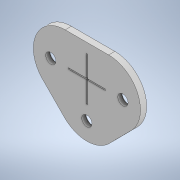
# Autodesk Inventor part: Cover
Saved by Autodesk Inventor 2021 (Build 250183000, 183)
## iProperties
Created: 2021-05-18
Part Number: Cover
Material: Generic
Document SubType Name: Modeling
Designer: Timo
Density: 1 g/cm^3
Appearance: Default
Mass: 1.07498 g
Surface Area: 14.5112 cm^2
Volume: 1.07498 cm^3
Author: Timo
Autodesk Inventor part; units mm, degrees
ref_plane "YZ Plane" through (0, 0, 0) normal (1, 0, 0) x (0, 1, 0)
ref_plane "XZ Plane" through (0, 0, 0) normal (0, 1, 0) x (-1, 0, 0)
ref_plane "XY Plane" through (0, 0, 0) normal (0, 0, 1) x (1, 0, 0)
sketch "Sketch1" plane through (0, 0, 0) normal (0, 0, 1) x (1, 0, 0)
  circle A0 centre (0, 0) radius 6.5 construction
  ellipse E0 centre (0, -17.162) end of major axis (0, -11.841) minor radius 5 construction
  line L0 (0, -44.4052) -> (0, 16.7342) projected
  ellipse E1 centre (0, -19.38) end of major axis (0, -14.059) minor radius 5 construction
  line L1 (0, -17.162) -> (0, -19.38) construction
  line L2 (-6, -17.162) -> (-6, -19.38)
  line L3 (6, -19.38) -> (6, -17.162)
  arc A1 (6, -17.162) -> (-6, -17.162) centre (0, -17.162) ccw
  arc A2 (-6, -19.38) -> (6, -19.38) centre (0, -19.38) ccw
  circle A3 centre (0, 0) radius 8 construction
  circle A4 centre (11.65, -18.271) radius 1.65
  line L4 (11.65, -18.271) -> (6, -18.271) construction
  circle A5 centre (-11.65, -18.271) radius 1.65
  line L5 (7.029, -18.271) -> (-7.029, -18.271) construction
  line L6 (7.029, -28.542) -> (-7.029, -28.542)
  line L7 (-7.029, -8) -> (7.029, -8)
  arc A6 (7.029, -28.542) -> (7.029, -8) centre (7.029, -18.271) ccw
  arc A7 (-7.029, -8) -> (-7.029, -28.542) centre (-7.029, -18.271) ccw
  circle A8 centre (0, -30) radius 1.65
  circle A9 centre (0, -25.4) radius 10.271
  line L8 (-14.3428, -25.4822) -> (-7.3138, -32.6112)
  line L9 (7.3138, -32.6112) -> (14.3428, -25.4822)
  line L10 (11.65, -18.271) -> (0, 0) construction
  point P0 (0, -18.271)
  point P1 (0, -8)
  point P2 (-0.7725, -28.542)
  point P3 (0.7725, -28.542)
  dimension "d7" = 5
  dimension "d8" = 5.321
  dimension "d10" = 5.321
  dimension "d11" = 5
  dimension "d0" = 13
  dimension "d9" = 17.162
  dimension "d12" = 2.218
  dimension "d13" = 12
  dimension "d14" = 1.5
  dimension "d15" = 3.3
  dimension "d16" = 4
  dimension "d17" = 4
  dimension "d18" = 3.3
  dimension "d19" = 4
  dimension "d50" = 3.3
  dimension "d51" = 30
  dimension "d52" = 4.6
  dimension "d54" = 21.6691
  dimension "d55" = 32.523
  constraints: 24 end point, 12 point on circle, 12 tangent, 9 centre point, 5 point on line, 4 midpoint, 2 parallel, 1 coincident, 1 collinear, 1 equal radius, 1 horizontal, 1 perpendicular, 1 vertical alignment, 6 other
  measures "d0" diameter of A0
  measures "d9" distance of L10.end L1.start
  measures "d12" distance of L1.start L1.end
  measures "d13" diameter of A2
  measures "d15" diameter of A4
  measures "d16" distance edge to line of A4 L3
  measures "d17" distance edge to line of A5 L2
  measures "d18" diameter of A5
  measures "d50" diameter of A8
  measures "d51" distance of point (0, 0) A8.centre
  measures "d52" distance of A9.centre A8.centre
  measures "d54" distance of point (0, 0) L4.start
  measures "d55" angle of L10 L0
extrude "Extrusion3" add sketch "Sketch1" along normal blind 2 contours A9 A7 L6 A8 L0 | L0 A8 L6 A6 A9 | L8 A7 A9 | A9 A6 L9 | L6 A7 A9 A1 L2 A2 L0 A8 | A7 L7 L0 A1 A9 | A9 A1 L0 L7 A6 | A6 L6 A8 L0 A2 L3 A1 A9
sketch "Sketch4" plane through (0, 0, 2) normal (0, 0, 1) x (1, 0, 0)
  line L0 (6, -17.162) -> (6, -19.38) projected
  line L1 (6, -18.471) -> (-6, -18.471)
  line L2 (6, -18.071) -> (-6, -18.071)
  line L3 (6, -18.271) -> (-6, -18.271) construction
  line L4 (-6, -19.38) -> (-6, -17.162) construction
  line L5 (0.2, -11.1653) -> (0.2, -25.3767)
  arc A0 (6, -17.162) -> (-6, -17.162) centre (0, -17.162) ccw projected
  line L6 (-0.2, -11.1653) -> (-0.2, -25.3767)
  line L7 (0, -42.8052) -> (0, 7.1342) projected
  arc A1 (-6, -19.38) -> (6, -19.38) centre (0, -19.38) ccw projected
  arc A2 (-7.029, -8) -> (-14.3428, -25.4822) centre (-7.029, -18.271) ccw projected
  arc A3 (14.3428, -25.4822) -> (7.029, -8) centre (7.029, -18.271) ccw projected
  line L8 (7.029, -8) -> (-7.029, -8) projected
  arc A4 (6, -17.162) -> (-6, -17.162) centre (0, -17.162) ccw projected
  line L9 (6, -17.162) -> (6, -19.38) projected
  arc A5 (-6, -19.38) -> (6, -19.38) centre (0, -19.38) ccw projected
  line L10 (-6, -19.38) -> (-6, -17.162) projected
  circle A6 centre (-11.65, -18.271) radius 1.65 projected
  circle A7 centre (11.65, -18.271) radius 1.65 projected
  line L11 (-14.3428, -25.4822) -> (-7.3138, -32.6112) projected
  arc A8 (-7.3138, -32.6112) -> (7.3138, -32.6112) centre (0, -25.4) ccw projected
  line L12 (7.3138, -32.6112) -> (14.3428, -25.4822) projected
  point P0 (0, 0)
  point P1 (-6, -18.471)
  point P2 (-0.2, -18.471)
  point P3 (0.2, -18.471)
  point P4 (0.2, -18.071)
  point P5 (-6, -18.071)
  point P6 (-0.2, -18.071)
  dimension "d22" = 0.4
  dimension "d23" = 0.4
  constraints: 10 end point, 4 point on circle, 4 point on line, 2 horizontal, 2 midpoint, 2 vertical, 2 other
  measures "d22" distance between parallel lines of L1 L2
  measures "d23" distance between parallel lines of L6 L5
extrude "Extrusion4" add sketch "Sketch4" against normal blind 1.5 contours L0 L2 L5 A0 | L0 A1 L5 L1 | L6 L2 L10 A0 | L6 A1 L10 L1
chamfer "Chamfer1" distance 0.7 angle 45 5 edges at (10, -18.271, 0) (-13.3, -18.271, 0) (-0.8509, -31.4137, 0) (0, -28.35, 0) (1.4137, -29.1491, 0)
sketch "Sketch5" plane through (0, 0, 0) normal (0, 0, -1) x (-1, 0, 0)
  line L0 (-19.5, -6.271) -> (19.5, -6.271)
  line L1 (19.5, -6.271) -> (19.5, -30.271)
  line L2 (19.5, -30.271) -> (-19.5, -30.271)
  line L3 (-19.5, -30.271) -> (-19.5, -6.271)
  line L4 (-19.5, -6.271) -> (19.5, -30.271) construction
  line L5 (19.5, -6.271) -> (-19.5, -30.271) construction
  line L6 (7.029, -28.542) -> (-7.029, -28.542) projected
  line L7 (-7.029, -8) -> (7.029, -8) projected
  arc A0 (14.3428, -25.4822) -> (7.029, -8) centre (7.029, -18.271) ccw projected
  line L8 (0, -42.8052) -> (0, 7.1342) projected
  line L9 (6, -18.471) -> (0.2, -18.471) construction
  line L10 (-0.2, -18.071) -> (0.2, -18.471) construction
  line L11 (-0.2, -25.3767) -> (-0.2, -18.471) construction
  line L12 (-0.2, -18.471) -> (0.2, -18.071) construction
  line L13 (19.5, -30.271) -> (15.6547, -34.171)
  line L14 (15.6547, -34.171) -> (-15.6547, -34.171)
  line L15 (-15.6547, -34.171) -> (-19.5, -30.271)
  line L16 (-7.3138, -32.6112) -> (-14.3428, -25.4822) projected
  line L17 (14.3428, -25.4822) -> (7.3138, -32.6112) projected
  arc A1 (-7.3138, -32.6112) -> (7.3138, -32.6112) centre (0, -25.4) ccw projected
  point P0 (0, 0)
  point P1 (0, -18.271)
  point P2 (0, -18.271)
  point P3 (0, -18.271)
  dimension "d36" = 24
  dimension "d37" = 39
  dimension "d53" = 1.5
  constraints: 22 end point, 5 midpoint, 4 parallel, 2 horizontal, 2 perpendicular, 1 point on line
  measures "d36" distance of L0.end L1.end
  measures "d37" distance of L1.end L2.end
  measures "d53" distance edge to line of A1 L14
sketch "Sketch8" plane through (0, 0, 2) normal (0, 0, 1) x (1, 0, 0)
  line L0 (-0.2, -11.1653) -> (-0.2, -18.071) projected
  line L1 (-0.2, -18.071) -> (-6, -18.071) projected
  line L2 (-6, -18.071) -> (-6, -18.471) projected
  line L3 (-6, -18.471) -> (-0.2, -18.471) projected
  line L4 (-0.2, -18.471) -> (-0.2, -25.3767) projected
  arc A0 (-0.2, -25.3767) -> (0.2, -25.3767) centre (0, -19.38) ccw projected
  line L5 (0.2, -25.3767) -> (0.2, -18.471) projected
  line L6 (0.2, -18.471) -> (6, -18.471) projected
  line L7 (6, -18.471) -> (6, -18.071) projected
  line L8 (6, -18.071) -> (0.2, -18.071) projected
  line L9 (0.2, -18.071) -> (0.2, -11.1653) projected
  arc A1 (0.2, -11.1653) -> (-0.2, -11.1653) centre (0, -17.162) ccw projected
  line L10 (0.2, -18.471) -> (0.2, -25.3767)
  arc A2 (-0.2, -25.3767) -> (0.2, -25.3767) centre (0, -19.38) ccw
  line L11 (-0.2, -25.3767) -> (-0.2, -18.471)
  line L12 (-0.2, -18.471) -> (-6, -18.471)
  line L13 (-6, -18.471) -> (-6, -18.071)
  line L14 (-6, -18.071) -> (-0.2, -18.071)
  line L15 (-0.2, -18.071) -> (-0.2, -11.1653)
  arc A3 (0.2, -11.1653) -> (-0.2, -11.1653) centre (0, -17.162) ccw
  line L16 (0.2, -11.1653) -> (0.2, -18.071)
  line L17 (0.2, -18.071) -> (6, -18.071)
  line L18 (6, -18.071) -> (6, -18.471)
  line L19 (6, -18.471) -> (0.2, -18.471)
  line L20 (-0.2, -11.1653) -> (-0.2, -11.1653)
  arc A4 (0.2, -11.1653) -> (-0.2, -11.1653) centre (0, -17.162) ccw projected
  line L21 (0.2, -11.1653) -> (0.2, -11.1653)
  line L22 (0.2, -25.3767) -> (0.2, -25.3767)
  line L23 (-0.2, -25.3767) -> (-0.2, -25.3767)
  line L24 (-6, -18.471) -> (-6, -18.471)
  line L25 (-6, -18.071) -> (-6, -18.471) projected
  line L26 (-6, -18.071) -> (-6, -18.071)
  line L27 (6, -18.071) -> (6, -18.071)
  line L28 (6, -18.471) -> (6, -18.471)
  point P0 (0, 0)
  dimension "d47" = 0.4
  constraints: 36 end point, 8 point on circle, 8 point on line, 2 centre point, 2 perpendicular, 1 parallel, 1 vertical, 11 other
  measures "d47" distance between parallel lines of L11 L10
sketch "Sketch6" plane through (-6, 6.479, 2) normal (0, 0, 1) x (1, 0, 0)
  line L0 (5.25, 6.3119) -> (5.25, 0) projected
  line L1 (5.25, 0) -> (0, 0) projected
  line L2 (0, 0) -> (0, -1.5) projected
  line L3 (0, -1.5) -> (5.25, -1.5) projected
  line L4 (5.25, -1.5) -> (5.25, -7.8119) projected
  arc A0 (5.25, -7.8119) -> (6.75, -7.8119) centre (6, -1.859) ccw projected
  line L5 (6.75, -7.8119) -> (6.75, -1.5) projected
  line L6 (6.75, -1.5) -> (12, -1.5) projected
  line L7 (12, -1.5) -> (12, 0) projected
  line L8 (12, 0) -> (6.75, 0) projected
  line L9 (6.75, 0) -> (6.75, 6.3119) projected
  arc A1 (6.75, 6.3119) -> (5.25, 6.3119) centre (6, 0.359) ccw projected
  line L10 (6.5, -0.25) -> (11.75, -0.25)
  line L11 (11.75, -0.25) -> (11.75, -1.25)
  line L12 (11.75, -1.25) -> (6.5, -1.25)
  line L13 (6.5, -1.25) -> (6.5, -7.5872)
  arc A2 (5.5, -7.5872) -> (6.5, -7.5872) centre (6, -1.859) ccw
  line L14 (5.5, -7.5872) -> (5.5, -1.25)
  line L15 (5.5, -1.25) -> (0.25, -1.25)
  line L16 (0.25, -1.25) -> (0.25, -0.25)
  line L17 (0.25, -0.25) -> (5.5, -0.25)
  line L18 (5.5, -0.25) -> (5.5, 6.0872)
  arc A3 (6.5, 6.0872) -> (5.5, 6.0872) centre (6, 0.359) ccw
  line L19 (6.5, 6.0872) -> (6.5, -0.25)
  point P0 (6, -6.479)
  dimension "d41" = 0.25
  constraints: 20 end point, 4 point on circle, 2 centre point, 11 other
  measures "d41" distance between parallel lines of L8 L10
sketch "Sketch7" plane through (0, 0, 2) normal (0, 0, 1) x (1, 0, 0)
  line L0 (18.2501, 17.0189) -> (18.2501, 11.7049) construction
  line L1 (18.2501, 11.7049) -> (11.9326, 11.7049) construction
  line L2 (11.9326, 11.7049) -> (11.9326, 17.0189) construction
  line L3 (11.9326, 17.0189) -> (18.2501, 17.0189) construction
  line L4 (-15.246, -25.6115) -> (-15.246, -29.9114) construction
  line L5 (-15.246, -29.9114) -> (-18.746, -29.9114) construction
  line L6 (-18.746, -29.9114) -> (-18.746, -25.6115) construction
  line L7 (-18.746, -25.6115) -> (-15.246, -25.6115) construction
  point P0 (0, 0)
  constraints: 4 other
equation "\"d10\" = d8"
equation "\"d11\" = d7"
equation "\"d17\" = d16"
equation "\"d18\" = d15"
equation "\"d50\" = d15"
equation "\"d23\" = d22"
body "Solid2"
body "Solid3"
